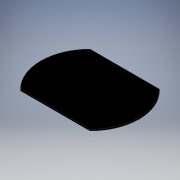
# Autodesk Inventor part: Gear Container Lid
Saved by Autodesk Inventor 2017 (Build 210142000, 142)
## iProperties
Created: 2018-12-13
Part Number: Gear Container Lid
Material: Generic
Document SubType Name: Modeling
Designer: Matt
Density: 1 g/cm^3
Appearance: Anodized - Black
Author: Matt
Autodesk Inventor part; units mm, degrees
ref_plane "YZ Plane" through (0, 0, 0) normal (1, 0, 0) x (0, 1, 0)
ref_plane "XZ Plane" through (0, 0, 0) normal (0, 1, 0) x (-1, 0, 0)
ref_plane "XY Plane" through (0, 0, 0) normal (0, 0, 1) x (1, 0, 0)
sketch "Sketch3" plane through (0, 0, 0) normal (0, 0, 1) x (1, 0, 0)
  line L0 (91.9239, 91.9239) -> (-91.9239, 91.9239)
  line L1 (-91.9239, 91.9239) -> (91.9239, 91.9239)
  arc A0 (91.9239, -91.9239) -> (91.9239, 91.9239) centre (0, 0) ccw
  arc A1 (91.9239, -91.9239) -> (91.9239, 91.9239) centre (91.9239, 0) ccw
  line L2 (91.9239, -91.9239) -> (-91.9239, -91.9239)
  arc A2 (-91.9239, 91.9239) -> (-91.9239, -91.9239) centre (0, 0) ccw
  arc A3 (-91.9239, 91.9239) -> (-91.9239, -91.9239) centre (-91.9239, 0) ccw
  dimension "d2" = 183.8478
  dimension "d3" = 183.8478
  constraints: 8 point on circle, 6 end point, 4 centre point, 1 collinear, 1 horizontal
  measures "d2" distance of L0.start L0.end
  measures "d3" distance between parallel lines of L2 L0
extrude "Extrusion2" add sketch "Sketch3" along normal blind 3.75 contours A0 L2 A2 L0
body "Solid2"
